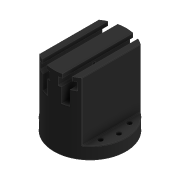
# Autodesk Inventor part: grippershape
Saved by Autodesk Inventor 2020.3 (Build 243373000, 373)
## iProperties
Created: 2020-05-25
Part Number: grippershape
Material: Generic
Document SubType Name: Modeling
Designer: Svend
Density: 1 g/cm^3
Appearance: Default
Author: Svend
Autodesk Inventor part; units mm, degrees
ref_plane "YZ Plane" through (0, 0, 0) normal (1, 0, 0) x (0, 1, 0)
ref_plane "XZ Plane" through (0, 0, 0) normal (0, 1, 0) x (-1, 0, 0)
ref_plane "XY Plane" through (0, 0, 0) normal (0, 0, 1) x (1, 0, 0)
ref_plane "Work Plane2" through (-6.6, -11, -70) normal (0, 0, -1) x (0, 1, 0)
ref_plane "Work Plane3" through (21.95, -1.9, -8.0264) normal (0, 0, 1) x (1, 0, 0)
ref_plane "Work Plane4" through (21.95, -1.9, -8.0264) normal (0, 0, 1) x (1, 0, 0)
sketch "Sketch3" plane through (21.95, -1.9, -8.0264) normal (0, 0, 1) x (1, 0, 0)
  line L0 (-6.75, 7.95) -> (-6.75, 1.35) projected
  line L1 (-6.75, 1.35) -> (-6.55, 1.15) projected
  line L2 (-6.55, 1.15) -> (-1.7, 1.15) projected
  line L3 (-1.7, 1.15) -> (-1.7, -12.85) projected
  line L4 (-4.0364, -12.85) -> (-4.0294, -12.85) projected
  line L5 (-2.65, -12.85) -> (-4.0294, -12.85) projected
  line L6 (-1.7, -12.85) -> (-2.65, -12.85) projected
  line L7 (-2.65, -12.85) -> (-2.65, -0.85) projected
  line L8 (-6.75, 7.95) -> (-6.55, 8.15) projected
  line L9 (-3.2, 8.15) -> (-6.55, 8.15) projected
  line L10 (-3.2, 12.75) -> (-3.2, 8.15) projected
  line L11 (-3.2, 12.75) -> (-3, 12.95) projected
  line L12 (3.1, 12.95) -> (-3, 12.95) projected
  line L13 (3.1, 12.95) -> (3.3, 12.75) projected
  line L14 (3.3, 8.15) -> (3.3, 12.75) projected
  line L15 (6.65, 8.15) -> (3.3, 8.15) projected
  line L16 (6.65, 8.15) -> (6.85, 7.95) projected
  line L17 (6.85, 1.35) -> (6.85, 7.95) projected
  line L18 (6.85, 1.35) -> (6.65, 1.15) projected
  line L19 (1.8, 1.15) -> (6.65, 1.15) projected
  line L20 (1.8, -12.65) -> (1.8, 1.15) projected
  line L21 (1.8, -12.85) -> (1.8, -12.65) projected
  line L22 (-1.7, -12.85) -> (1.8, -12.85) projected
  line L23 (-4.0294, -12.85) -> (-4.125, 1.15)
  line L24 (-7.05, 1.2257) -> (-7.05, 8.0743)
  line L25 (-7.05, 8.0743) -> (-6.6743, 8.45)
  line L26 (-6.6743, 8.45) -> (-3.5, 8.45)
  line L27 (-3.5, 8.45) -> (-3.5, 12.8743)
  line L28 (-3.5, 12.8743) -> (-3.1243, 13.25)
  line L29 (-3.1243, 13.25) -> (3.2243, 13.25)
  line L30 (3.2243, 13.25) -> (3.6, 12.8743)
  line L31 (3.6, 12.8743) -> (3.6, 8.45)
  line L32 (3.6, 8.45) -> (6.7743, 8.45)
  line L33 (6.7743, 8.45) -> (7.15, 8.0743)
  line L34 (7.15, 8.0743) -> (7.15, 1.2257)
  line L35 (7.15, 1.2257) -> (6.7743, 0.85)
  line L36 (6.7743, 0.85) -> (2.1, 0.85)
  line L37 (2.1, 0.85) -> (2.1, -12.65)
  line L38 (2.1, -12.65) -> (2.1, -13.15)
  line L39 (2.1, -13.15) -> (-2, -13.15)
  line L40 (-2, -13.15) -> (-2, 0.85)
  line L41 (-2, 0.85) -> (-6.6743, 0.85)
  line L42 (-6.6743, 0.85) -> (-7.05, 1.2257)
  line L43 (-4.1273, -13.15) -> (-4.2253, 1.1991)
  line L44 (-2, -13.15) -> (-4.1273, -13.15)
  line L45 (-13.925, -1.05) -> (-8.025, -1.05) projected
  line L46 (-10.975, -1.05) -> (-10.975, -12.3939)
  line L47 (-15.2, 7.95) -> (-15.2, 1.35)
  line L48 (-15.2, 1.35) -> (-15.4, 1.15)
  line L49 (-15.4, 1.15) -> (-20.25, 1.15)
  line L50 (-20.25, 1.15) -> (-20.25, -12.85)
  line L51 (-17.9136, -12.85) -> (-17.9206, -12.85)
  line L52 (-19.3, -12.85) -> (-17.9206, -12.85)
  line L53 (-20.25, -12.85) -> (-19.3, -12.85)
  line L54 (-19.3, -12.85) -> (-19.3, -0.85)
  line L55 (-15.2, 7.95) -> (-15.4, 8.15)
  line L56 (-18.75, 8.15) -> (-15.4, 8.15)
  line L57 (-18.75, 12.75) -> (-18.75, 8.15)
  line L58 (-18.75, 12.75) -> (-18.95, 12.95)
  line L59 (-25.05, 12.95) -> (-18.95, 12.95)
  line L60 (-25.05, 12.95) -> (-25.25, 12.75)
  line L61 (-25.25, 8.15) -> (-25.25, 12.75)
  line L62 (-28.6, 8.15) -> (-25.25, 8.15)
  line L63 (-28.6, 8.15) -> (-28.8, 7.95)
  line L64 (-28.8, 1.35) -> (-28.8, 7.95)
  line L65 (-28.8, 1.35) -> (-28.6, 1.15)
  line L66 (-23.75, 1.15) -> (-28.6, 1.15)
  line L67 (-23.75, -12.65) -> (-23.75, 1.15)
  line L68 (-23.75, -12.85) -> (-23.75, -12.65)
  line L69 (-20.25, -12.85) -> (-23.75, -12.85)
  line L70 (-17.9206, -12.85) -> (-17.825, 1.15)
  line L71 (-14.9, 1.2257) -> (-14.9, 8.0743)
  line L72 (-14.9, 8.0743) -> (-15.2757, 8.45)
  line L73 (-15.2757, 8.45) -> (-18.45, 8.45)
  line L74 (-18.45, 8.45) -> (-18.45, 12.8743)
  line L75 (-18.45, 12.8743) -> (-18.8257, 13.25)
  line L76 (-18.8257, 13.25) -> (-25.1743, 13.25)
  line L77 (-25.1743, 13.25) -> (-25.55, 12.8743)
  line L78 (-25.55, 12.8743) -> (-25.55, 8.45)
  line L79 (-25.55, 8.45) -> (-28.7243, 8.45)
  line L80 (-28.7243, 8.45) -> (-29.1, 8.0743)
  line L81 (-29.1, 8.0743) -> (-29.1, 1.2257)
  line L82 (-29.1, 1.2257) -> (-28.7243, 0.85)
  line L83 (-28.7243, 0.85) -> (-24.05, 0.85)
  line L84 (-24.05, 0.85) -> (-24.05, -12.65)
  line L85 (-24.05, -12.65) -> (-24.05, -13.15)
  line L86 (-24.05, -13.15) -> (-19.95, -13.15)
  line L87 (-19.95, -13.15) -> (-19.95, 0.85)
  line L88 (-19.95, 0.85) -> (-15.2757, 0.85)
  line L89 (-15.2757, 0.85) -> (-14.9, 1.2257)
  line L90 (-17.8227, -13.15) -> (-17.7247, 1.1991)
  line L91 (-19.95, -13.15) -> (-17.8227, -13.15)
  line L92 (-33.425, 12.25) -> (11.575, 12.25)
  line L93 (11.575, 12.25) -> (11.575, -57.75)
  line L94 (11.575, -57.75) -> (-33.425, -57.75)
  line L95 (-33.425, -57.75) -> (-33.425, 12.25)
  point P0 (-21.95, 1.9)
  point P1 (-10.925, -52.6184)
  point P2 (-10.925, -57.75)
  point P3 (-3.5, 12.25)
  point P4 (-18.45, 12.25)
  point P5 (-17.727, 0.85)
  point P6 (-25.55, 12.25)
  point P7 (3.6, 12.25)
  point P8 (-4.223, 0.85)
  dimension "d18" = 0.3
  dimension "d19" = 0.1
  dimension "d20" = 1
  dimension "d21" = 45
  dimension "d22" = 70
  constraints: 144 end point, 45 symmetric about line, 3 midpoint, 3 parallel, 2 horizontal, 1 perpendicular, 1 vertical, 1 vertical alignment, 18 other
  measures "d18" distance between parallel lines of L0 L24
  measures "d19" distance between parallel lines of L23 L43
  measures "d20" distance between parallel lines of L76 L92
  measures "d21" distance of L93.end L94.end
  measures "d22" distance between parallel lines of L92 L94
extrude "Extrusion2" add sketch "Sketch3" against normal blind 70 contours L43 L44 L39 L38 L37 L36 L35 L34 L33 L32 L31 L92 L93 L94 L95 L78 L79 L80 L81 L82 L83 L84 L85 L86 L91 L90 L88 L89 L71 L72 L73 L74 L27 L26 L25 L24 L42 L41
sketch "Sketch4" plane through (-11.475, -59.65, -8.0264) normal (0, -1, 0) x (1, 0, 0)
  line L0 (0, 0) -> (45, 0) projected
  line L1 (0, 0) -> (0, -70) projected
  line L2 (45, -70) -> (0, -70) projected
  line L3 (45, 0) -> (45, -70) projected
  circle A0 centre (22.5, -35) radius 9
  point P0 (11.475, 8.0264)
  point P1 (22.5, 0)
  point P2 (45, -35)
  dimension "d25" = 18
  constraints: 2 midpoint, 1 centre point, 1 horizontal alignment, 1 vertical alignment
  measures "d25" diameter of A0
ref_plane "Work Plane5" through (1.75, -2.8, -26.5932) normal (0, 1, 0) x (0, 0, 1)
extrude "Extrusion3" cut sketch "Sketch4" against normal blind 57.25 contours A0
sketch "Sketch5" plane through (-11.475, -59.65, -8.0264) normal (0, -1, 0) x (1, 0, 0)
  circle A0 centre (22.5, -35) radius 9 projected
  circle A1 centre (22.5, -35) radius 4
  point P0 (11.475, 8.0264)
  dimension "d28" = 8
  constraints: 1 centre point, 1 coincident
  measures "d28" diameter of A1
extrude "Extrusion4" cut sketch "Sketch5" against normal blind 61 contours A1
ref_plane "Work Plane6" through (1.2787, -51.0682, -52.9264) normal (0, 0, -1) x (0, 1, 0)
sketch "Sketch8" plane through (-11.475, -59.65, -8.0264) normal (0, -1, 0) x (1, 0, 0)
  circle A0 centre (22.5, -35) radius 9 projected
  circle A1 centre (22.5, -35) radius 9 projected
  line L0 (0, 0) -> (45, 0) projected
  line L1 (0, 0) -> (0, -70) projected
  line L2 (45, -70) -> (0, -70) projected
  line L3 (45, 0) -> (45, -70) projected
  arc A2 (26.375, -34.0078) -> (18.525, -34.5535) centre (22.5, -35) ccw projected
  circle A3 centre (22.5, -35) radius 35
  point P0 (11.475, 8.0264)
  point P1 (45, -8.1905)
  point P2 (45, -61.8095)
  point P3 (0, -61.8095)
  point P4 (0, -8.1905)
  point P5 (22.5, -70)
  point P6 (22.5, 0)
  constraints: 1 centre point, 1 coincident, 1 tangent
extrude "Extrusion10" cut sketch "Sketch8" against normal through all contours L0 A3 L1 | L0 L3 A3 | A3 L2 L1 | L3 L2 A3
ref_plane "Work Plane7" through (10.975, -59.9, -43.0264) normal (0, -1, 0) x (1, 0, 0)
sketch "Sketch10" plane through (10.975, -59.9, -43.0264) normal (0, -1, 0) x (1, 0, 0)
  line L0 (29.6, 9.9) -> (-9, 9.9) projected
  arc A0 (-9, 9.9) -> (-10, 8.9) centre (-9, 8.9) ccw projected
  line L1 (-10, 8.9) -> (-10, -8.9) projected
  arc A1 (30.6, 8.9) -> (29.6, 9.9) centre (29.6, 8.9) ccw projected
  line L2 (30.6, -8.9) -> (30.6, 8.9) projected
  arc A2 (29.6, -9.9) -> (30.6, -8.9) centre (29.6, -8.9) ccw projected
  line L3 (-9, -9.9) -> (29.6, -9.9) projected
  arc A3 (-10, -8.9) -> (-9, -9.9) centre (-9, -8.9) ccw projected
  line L4 (-10, 8.9) -> (-10, -8.9) projected
  line L5 (-10.2, -12) -> (-10.2, 30.5)
  line L6 (-10.2, 30.5) -> (10.2, 30.5)
  line L7 (10.2, 30.5) -> (10.2, -12)
  line L8 (10.2, -12) -> (-10.2, -12)
  circle A4 centre (0, 0) radius 9 projected
  circle A5 centre (0.05, 0) radius 9 projected
  arc A6 (22.55, 26.8095) -> (-22.45, 26.8095) centre (0.05, 0) ccw projected
  line L9 (-22.45, 26.8095) -> (-22.45, -26.8095) projected
  arc A7 (-22.45, -26.8095) -> (22.55, -26.8095) centre (0.05, 0) ccw projected
  line L10 (22.55, 26.8095) -> (22.55, -26.8095) projected
  point P0 (-10.975, 43.0264)
  point P1 (0, -12)
  dimension "d45" = 20.4
  dimension "d46" = 12
  dimension "d47" = 30.5
  constraints: 8 end point, 2 parallel, 1 midpoint, 1 perpendicular
  measures "d45" distance between parallel lines of L7 L5
  measures "d46" distance from line of L8 A4.centre
  measures "d47" distance from line of L6 A4.centre
extrude "Extrusion12" cut sketch "Sketch10" against normal blind 43 contours L7 L3 A3 L1 A0 L0 | L0 A0 L1 A3 L3 L7 L8 L5 L6 | A4 A5 | A4 A5 | A5 A4
sketch "Sketch11" plane through (0.775, -59.65, -55.0264) normal (0, 0, 1) x (1, 0, 0)
  line L0 (20.4, 0) -> (0, 0) projected
  line L1 (20.4, 0) -> (20.4, 42.75) projected
  line L2 (20.4, 42.75) -> (0, 42.75) projected
  line L3 (0, 0) -> (0, 42.75) projected
  line L4 (5.7, 15) -> (14.7, 15)
  line L5 (14.7, 15) -> (14.7, 8)
  line L6 (14.7, 8) -> (5.7, 8)
  line L7 (5.7, 8) -> (5.7, 15)
  point P0 (-32.8264, 59.9)
  point P1 (10.2, 8)
  point P2 (10.2, 0)
  dimension "d50" = 8
  dimension "d51" = 7
  dimension "d52" = 9
  constraints: 8 end point, 2 midpoint, 2 parallel, 1 horizontal, 1 perpendicular, 1 vertical alignment
  measures "d50" distance between parallel lines of L0 L6
  measures "d51" distance between parallel lines of L6 L4
  measures "d52" distance between parallel lines of L7 L5
extrude "Extrusion13" cut sketch "Sketch11" against normal through all contours L4 L5 L6 L7
fillet "Fillet10" radius 0.2 4 edges at (25.55, 10.35, -43.0264) (18.45, 10.35, -43.0264) (3.5, 10.35, -43.0264) (-3.6, 10.35, -43.0264)
chamfer "Chamfer5" distance 0.5 angle 45 6 edges at (20.0062, -15.05, -42.4455) (20.0062, -15.05, -43.6074) (19.2357, -15.05, -39.3407) (19.2357, -15.05, -46.7122) (2.025, -15.05, -43.0264) (7.025, -2.4, -43.0264)
fillet "Fillet11" radius 0.2 10 edges at (4.1256, -15.3001, -37.2473) (4.1703, -8.7525, -37.1943) (4.2137, -2.4, -43.0264) (4.1256, -15.3001, -48.8056) (4.1703, -8.7525, -48.8586) (17.7796, -8.7511, -48.9741) (17.8244, -15.3001, -48.9229) (17.7363, -2.4, -43.0264) (17.8244, -15.3001, -37.13) (17.7796, -8.7511, -37.0788)
extrude "Extrusion14" add sketch "Sketch8" against normal blind 13.15 contours L1 A3 | A3 L3
sketch "Sketch13" plane through (11.025, 10.35, -43.0264) normal (0, 1, 0) x (0.9999989, 0, 0.0014605)
  circle A0 centre (0, 0) radius 35 projected
  line L0 (22.5391, -26.7766) -> (22.4608, 26.8423) projected
  line L1 (-22.5391, 26.7766) -> (-22.4608, -26.8423) projected
  line L2 (20.5414, -28.3381) -> (20.4585, 28.398)
  arc A1 (22.4608, 26.8423) -> (14.6786, 31.7732) centre (0, 0) ccw projected
  arc A2 (-14.8713, 31.6835) -> (-22.5391, 26.7766) centre (0, 0) ccw projected
  line L3 (-20.5, 28.3681) -> (-20.5, -28.3681)
  point P0 (-10.9621, -43.0425)
  point P1 (20.4585, 28.398)
  dimension "d85" = 2
  dimension "d86" = 2
  constraints: 4 end point, 2 point on circle, 1 parallel, 1 vertical, 4 other
  measures "d85" distance between parallel lines of L0 L2
extrude "Extrusion15" cut sketch "Sketch13" against normal up to surface (56.85 mm away) contours L0 A0 L2 | A0 L1 L3
sketch "Sketch14" plane through (11.025, -59.65, -43.0264) normal (0, -1, 0) x (1, 0, 0)
  line L0 (10.15, -12) -> (-10.25, -12) projected
  line L1 (-10.25, -12) -> (-10.25, 30.5) projected
  line L2 (-10.25, 30.5) -> (10.15, 30.5) projected
  line L3 (10.15, 30.5) -> (10.15, -12) projected
  circle A0 centre (0, 0) radius 35 projected
  circle A1 centre (28, 0) radius 2.1
  arc A2 (-9, 0) -> (-9, 0) centre (0, 0) ccw projected
  circle A3 centre (24.2487, 14) radius 2.1
  circle A4 centre (14, 24.2487) radius 2.1
  circle A5 centre (0, 28) radius 2.1
  circle A6 centre (-14, 24.2487) radius 2.1
  circle A7 centre (-24.2487, 14) radius 2.1
  circle A8 centre (-28, 0) radius 2.1
  circle A9 centre (-24.2487, -14) radius 2.1
  circle A10 centre (-14, -24.2487) radius 2.1
  circle A11 centre (0, -28) radius 2.1
  circle A12 centre (14, -24.2487) radius 2.1
  circle A13 centre (24.2487, -14) radius 2.1
  point P0 (-11.025, 43.0264)
  dimension "d89" = 28
  dimension "d90" = 4.2
  dimension "d93" = 360
  constraints: 12 centre point, 1 horizontal alignment, 25 other
  measures "d89" distance of A2.centre A1.centre
  measures "d90" diameter of A1
extrude "Extrusion16" cut sketch "Sketch14" against normal through all contours A1 | A3 | A7 | A8 | A9 | A13
sketch "Sketch15" plane through (11.025, -59.65, -43.0264) normal (0, -1, 0) x (1, 0, 0)
  circle A0 centre (24.2487, -14) radius 2.1 projected
  circle A1 centre (-24.2487, 14) radius 2.1 projected
  circle A2 centre (28, 0) radius 2.1 projected
  circle A3 centre (-24.2487, -14) radius 2.1 projected
  circle A4 centre (-28, 0) radius 2.1 projected
  circle A5 centre (24.2487, 14) radius 2.1 projected
  line L0 (10.15, -12) -> (-10.25, -12) projected
  line L1 (-10.25, -12) -> (-10.25, 30.5) projected
  line L2 (-10.25, 30.5) -> (10.15, 30.5) projected
  line L3 (10.15, 30.5) -> (10.15, -12) projected
  circle A6 centre (0, 0) radius 35 projected
  point P0 (-11.025, 43.0264)
extrude "Extrusion17" cut sketch "Sketch15" against normal blind 1.15
fillet "Fillet12" radius 0.5 48 edges at (11.025, -58.5, -8.0264) (11.025, -58.5, -78.0264) (-23.975, -58.5, -43.0264) (46.025, -58.5, -43.0264) (33.1737, -58.5, -29.0264) (36.925, -58.5, -43.0264) (33.1737, -58.5, -57.0264) (-15.3237, -58.5, -57.0264) (-19.075, -58.5, -43.0264) (-15.3237, -58.5, -29.0264) (-10.5093, -46.5, -15.4352) (-10.469, -46.5, -70.6491) (-23.975, -46.5, -43.0264) (-11.2135, -46.5, -28.4191) (-11.2135, -46.5, -29.6338) (-15.3237, -46.5, -29.0264) (-19.075, -46.5, -43.0264) (-11.2135, -46.5, -56.4191) (-11.2135, -46.5, -57.6338) (-15.3237, -46.5, -57.0264) (-9.475, -46.5, -43.0564) (21.175, -58.5, -33.7764) (10.975, -58.5, -55.0264) (0.775, -58.5, -33.7764) (10.975, -58.5, -12.5264) (31.525, -46.5, -43.0264) (33.1737, -46.5, -29.0264) (35.881, -46.5, -31.0367) (35.881, -46.5, -27.0162) (36.925, -46.5, -43.0264) (33.1737, -46.5, -57.0264) (35.881, -46.5, -59.0367) (35.881, -46.5, -55.0162) (32.5391, -46.5, -15.4195) (32.5391, -46.5, -70.6334) (46.025, -46.5, -43.0264) (31.525, -18.075, -14.6583) (31.525, -18.075, -71.3946) (31.525, 10.35, -43.0264) (-9.475, 10.35, -43.0564) (-9.5164, -18.075, -14.6883) (-9.4335, -18.075, -71.4245) (10.975, -44.65, -55.0264) (10.975, -51.65, -55.0264) (10.9746, -44.65, -78.0264) (6.475, -48.15, -77.7294) (15.475, -48.15, -77.7424) (10.9746, -51.65, -78.0264)
sketch "Sketch16" plane through (11.025, -58.5, -43.0264) normal (0, -1, 0) x (1, 0, 0)
  arc A0 (-4.5549, -34.198) -> (4.4547, -34.2112) centre (0, 0) ccw projected
  arc A1 (4.45, -34.143) -> (4.4547, -34.2112) centre (4.95, -34.143) ccw projected
  line L0 (4.45, -12.5) -> (4.45, -34.143) projected
  line L1 (-4.55, -12.5) -> (4.45, -12.5) projected
  line L2 (-4.55, -12.5) -> (-4.55, -34.1284) projected
  arc A2 (-4.5549, -34.198) -> (-4.55, -34.1284) centre (-5.05, -34.1284) ccw projected
  line L3 (10.15, -12) -> (-10.25, -12) projected
  line L4 (-4.55, -12.5) -> (-4.55, -34.1284) projected
  line L5 (4.45, -12) -> (-4.55, -12)
  line L6 (-4.55, -12) -> (-4.55, -27)
  line L7 (-4.55, -27) -> (4.45, -27)
  line L8 (4.45, -27) -> (4.45, -12)
  point P0 (-11.025, 43.0264)
  point P1 (-4.55, -27)
  point P2 (4.45, -27)
  point P3 (4.45, -12.5)
  point P4 (-4.55, -12)
  dimension "d100" = 15
  constraints: 8 end point, 2 collinear, 2 parallel, 2 point on line, 1 horizontal, 1 perpendicular
  measures "d100" distance of L6.end L5.end
extrude "Extrusion18" cut sketch "Sketch16" against normal up to surface (13.85 mm away) contours L2 L1 L0 L7 | L6 L3 L8 L1
sketch "Sketch17" plane through (11.025, -58.5, -43.0264) normal (0, -1, 0) x (1, 0, 0)
  line L0 (4.45, -12.5) -> (4.45, -27) projected
  line L1 (4.45, -27) -> (-4.55, -27) projected
  line L2 (-4.55, -27) -> (-4.55, -12.5) projected
  line L3 (-10.75, -12.5) -> (-4.55, -12.5) projected
  line L4 (-10.75, 31) -> (-10.75, -12.5) projected
  line L5 (10.65, 31) -> (-10.75, 31) projected
  line L6 (10.65, -12.5) -> (10.65, 31) projected
  line L7 (4.45, -12.5) -> (10.65, -12.5) projected
  circle A0 centre (-28, 0) radius 2.6 projected
  circle A1 centre (24.2487, -14) radius 2.6 projected
  circle A2 centre (24.2487, 14) radius 2.6 projected
  circle A3 centre (0, 0) radius 34.5 projected
  circle A4 centre (28, 0) radius 2.6 projected
  circle A5 centre (-24.2487, -14) radius 2.6 projected
  circle A6 centre (-24.2487, 14) radius 2.6 projected
  line L8 (-10.75, -12.5) -> (-4.55, -12.5) projected
  line L9 (5.95, -35) -> (-6.05, -35)
  line L10 (-6.05, -35) -> (-6.05, -12.5)
  line L11 (-6.05, -12.5) -> (5.95, -12.5)
  line L12 (5.95, -12.5) -> (5.95, -35)
  circle A7 centre (0, 0) radius 35 projected
  line L13 (7.7, -29.2) -> (-7.7, -29.2)
  line L14 (-7.7, -29.2) -> (-7.7, -27)
  line L15 (-7.7, -27) -> (7.7, -27)
  line L16 (7.7, -27) -> (7.7, -29.2)
  line L17 (10.15, -12) -> (4.45, -12) projected
  line L18 (4.45, -12) -> (-4.55, -12) projected
  line L19 (-4.55, -12) -> (-10.25, -12) projected
  line L20 (5.95, -12.5) -> (5.95, -12)
  line L21 (-6.05, -12.5) -> (-6.05, -12)
  point P0 (-11.025, 43.0264)
  point P1 (-0.05, -35)
  point P2 (-0.05, -27)
  point P3 (0, -29.2)
  point P4 (-6.05, -29.2)
  point P5 (-6.05, -33.9654)
  point P6 (5.95, -33.983)
  point P7 (5.95, -29.2)
  point P8 (5.95, -27)
  point P9 (-6.05, -27)
  point P10 (5.95, -34.4905)
  point P11 (-6.05, -34.4731)
  dimension "d104" = 12
  dimension "d105" = 15.4
  dimension "d106" = 2.2
  constraints: 20 end point, 4 parallel, 4 perpendicular, 3 midpoint, 3 point on line, 2 horizontal, 2 vertical alignment, 1 collinear, 1 tangent
  measures "d104" distance between parallel lines of L12 L10
  measures "d105" distance between parallel lines of L16 L14
  measures "d106" distance between parallel lines of L1 L13
extrude "Extrusion19" cut sketch "Sketch17" against normal blind 15.5 contours L7 L12 L15 L0 | L11 L3 L21 L19 L18 L17 L20 L7 | L0 L1 L2 L11 | L15 L12 L13 L10 L1 | L2 L15 L10 L3 | L15 L16 L13 L12 | L10 L13 L14 L15 | L12 A3 L10 L13 | L12 A7 L10 A3 picked at (3.9619, -34.4002)
sketch "Sketch18" plane through (0.775, -16.9, -55.0264) normal (0, 0, 1) x (1, 0, 0)
  line L0 (4.2, -41.1) -> (4.2, -26.1) projected
  line L1 (4.2, -26.1) -> (16.2, -26.1) projected
  line L2 (16.2, -26.1) -> (16.2, -41.1) projected
  arc A0 (16.2, -33.6) -> (4.2, -33.6) centre (10.2, -33.6) ccw
  point P0 (-0.775, 16.9)
  constraints: 2 midpoint, 2 point on circle, 2 tangent, 1 centre point
extrude "Extrusion20" add sketch "Sketch18" against normal up to surface (15 mm away)
sketch "Sketch19" plane through (3.325, -58.5, -72.2264) normal (0, 0, 1) x (1, 0, 0)
  line L0 (0, 0) -> (1.65, 0) projected
  line L1 (0, 0) -> (0, 15.5) projected
  line L2 (0, 15.5) -> (15.4, 15.5) projected
  line L3 (15.4, 0) -> (15.4, 15.5) projected
  line L4 (13.65, 0) -> (15.4, 0) projected
  line L5 (13.65, 0) -> (13.65, 8) projected
  arc A0 (13.65, 8) -> (1.65, 8) centre (7.65, 8) ccw projected
  line L6 (1.65, 0) -> (1.65, 8) projected
  line L7 (-1.1, 8) -> (-1.1, 0)
  line L8 (42.2, 0) -> (-26.8, 0) projected
  line L9 (16.4, 8) -> (16.4, 0)
  arc A1 (16.4, 8) -> (-1.1, 8) centre (7.65, 8) ccw
  point P0 (-3.325, 58.5)
  point P1 (15.4, 12.062)
  point P2 (0, 12.2474)
  point P3 (16.4, 0)
  constraints: 4 end point, 2 point on circle, 2 tangent, 2 vertical, 1 centre point, 1 coincident, 1 point on line
extrude "Extrusion21" cut sketch "Sketch19" against normal up to surface contours L1 A1 L2 L3 L4 L5 A0 L6 L0 | L8 L7 A1 L1 | A1 L2 | L3 A1 L9 L8 round surface about axis through (11.025, -59.65, -43.0264) along (0, 1, 0) radius 35 far side no
sketch "Sketch20" plane through (16.975, -43, -72.2264) normal (0, 0, 1) x (1, 0, 0)
  line L0 (0, -1.1311) -> (0, 0) projected
  line L1 (0, 0) -> (-1.4931, 0) projected
  line L2 (-10.5069, 0) -> (-12, 0) projected
  line L3 (-12, 0) -> (-12, -1.1311) projected
  line L4 (2.75, -15) -> (-14.75, -15) projected
  line L5 (8.775, 53.35) -> (14.05, 53.35) projected
  line L6 (8.575, 49.55) -> (8.575, 53.15) projected
  line L7 (11.7493, 49.55) -> (8.575, 49.55) projected
  line L8 (12.125, 49.1743) -> (11.7493, 49.55) projected
  line L9 (12.125, 42.3257) -> (12.125, 49.1743) projected
  line L10 (11.7493, 41.95) -> (12.125, 42.3257) projected
  line L11 (7.075, 41.95) -> (11.7493, 41.95) projected
  line L12 (7.075, 27.95) -> (7.075, 41.95) projected
  line L13 (0.8477, 27.95) -> (7.075, 27.95) projected
  line L14 (0.752, 41.95) -> (0.8477, 27.95) projected
  line L15 (-1.6993, 41.95) -> (0.752, 41.95) projected
  line L16 (-2.075, 42.3257) -> (-1.6993, 41.95) projected
  line L17 (-2.075, 49.1743) -> (-2.075, 42.3257) projected
  line L18 (-1.6993, 49.55) -> (-2.075, 49.1743) projected
  line L19 (1.475, 49.55) -> (-1.6993, 49.55) projected
  line L20 (1.475, 53.15) -> (1.475, 49.55) projected
  line L21 (-13.275, 53.35) -> (1.275, 53.35) projected
  line L22 (-13.475, 49.55) -> (-13.475, 53.15) projected
  line L23 (-10.3007, 49.55) -> (-13.475, 49.55) projected
  line L24 (-9.925, 49.1743) -> (-10.3007, 49.55) projected
  line L25 (-9.925, 42.3257) -> (-9.925, 49.1743) projected
  line L26 (-10.3007, 41.95) -> (-9.925, 42.3257) projected
  line L27 (-12.752, 41.95) -> (-10.3007, 41.95) projected
  line L28 (-12.8477, 27.95) -> (-12.752, 41.95) projected
  line L29 (-19.075, 27.95) -> (-12.8477, 27.95) projected
  line L30 (-19.075, 41.95) -> (-19.075, 27.95) projected
  line L31 (-23.7493, 41.95) -> (-19.075, 41.95) projected
  line L32 (-24.125, 42.3257) -> (-23.7493, 41.95) projected
  line L33 (-24.125, 49.1743) -> (-24.125, 42.3257) projected
  line L34 (-23.7493, 49.55) -> (-24.125, 49.1743) projected
  line L35 (-20.575, 49.55) -> (-23.7493, 49.55) projected
  line L36 (-20.575, 53.15) -> (-20.575, 49.55) projected
  line L37 (-25.9919, 53.35) -> (-20.775, 53.35) projected
  line L38 (-26.2815, -3) -> (-26.2815, 53.2574) projected
  line L39 (-27.2138, -4) -> (-27.2949, -4) projected
  line L40 (-26.1982, 53.2574) -> (-26.1982, -3) projected
  line L41 (-20.775, 53.35) -> (-25.908, 53.35) projected
  line L42 (-20.575, 49.55) -> (-20.575, 53.15) projected
  line L43 (-23.7493, 49.55) -> (-20.575, 49.55) projected
  line L44 (-24.125, 49.1743) -> (-23.7493, 49.55) projected
  line L45 (-24.125, 42.3257) -> (-24.125, 49.1743) projected
  line L46 (-23.7493, 41.95) -> (-24.125, 42.3257) projected
  line L47 (-19.075, 41.95) -> (-23.7493, 41.95) projected
  line L48 (-19.075, 27.95) -> (-19.075, 41.95) projected
  line L49 (-12.8477, 27.95) -> (-19.075, 27.95) projected
  line L50 (-12.752, 41.95) -> (-12.8477, 27.95) projected
  line L51 (-10.3007, 41.95) -> (-12.752, 41.95) projected
  line L52 (-9.925, 42.3257) -> (-10.3007, 41.95) projected
  line L53 (-9.925, 49.1743) -> (-9.925, 42.3257) projected
  line L54 (-10.3007, 49.55) -> (-9.925, 49.1743) projected
  line L55 (-13.475, 49.55) -> (-10.3007, 49.55) projected
  line L56 (-13.475, 53.15) -> (-13.475, 49.55) projected
  line L57 (1.275, 53.35) -> (-13.275, 53.35) projected
  line L58 (1.475, 49.55) -> (1.475, 53.15) projected
  line L59 (-1.6993, 49.55) -> (1.475, 49.55) projected
  line L60 (-2.075, 49.1743) -> (-1.6993, 49.55) projected
  line L61 (-2.075, 42.3257) -> (-2.075, 49.1743) projected
  line L62 (-1.6993, 41.95) -> (-2.075, 42.3257) projected
  line L63 (0.752, 41.95) -> (-1.6993, 41.95) projected
  line L64 (0.8477, 27.95) -> (0.752, 41.95) projected
  line L65 (7.075, 27.95) -> (0.8477, 27.95) projected
  line L66 (7.075, 41.95) -> (7.075, 27.95) projected
  line L67 (11.7493, 41.95) -> (7.075, 41.95) projected
  line L68 (12.125, 42.3257) -> (11.7493, 41.95) projected
  line L69 (12.125, 49.1743) -> (12.125, 42.3257) projected
  line L70 (11.7493, 49.55) -> (12.125, 49.1743) projected
  line L71 (8.575, 49.55) -> (11.7493, 49.55) projected
  line L72 (8.575, 53.15) -> (8.575, 49.55) projected
  line L73 (14.05, 53.35) -> (8.775, 53.35) projected
  line L74 (14.3399, -3) -> (14.3399, 53.2574) projected
  line L75 (15.3543, -4) -> (15.3543, -4) projected
  line L76 (14.3399, 53.2574) -> (14.3399, -3) projected
  circle A0 centre (-6, -7.5) radius 8.75
  line L77 (2.75, -15) -> (2.75, -7.5) projected
  line L78 (-14.75, -7.5) -> (-14.75, -15) projected
  point P0 (-16.975, 43)
  point P1 (-10.5069, 0)
  point P2 (-1.4931, 0)
  point P3 (0, -1.1311)
  constraints: 1 centre point, 1 horizontal alignment, 20 other
extrude "Extrusion22" add sketch "Sketch20" against normal up to surface contours A0 L1 L0 | A0 L3 L2 round surface about axis through (11.025, -59.65, -43.0264) along (0, 1, 0) radius 35 far side no
sketch "Sketch21" plane through (11.025, -43, -43.0264) normal (0, -1, 0) x (1, 0, 0)
  line L0 (-4.5569, -29.2) -> (-7.7, -29.2) projected
  line L1 (-4.5569, -29.2) -> (4.4569, -29.2) projected
  line L2 (4.4569, -29.2) -> (7.7, -29.2) projected
  line L3 (7.7, -27) -> (7.7, -29.2) projected
  line L4 (-7.7, -27) -> (7.7, -27) projected
  line L5 (-7.7, -29.2) -> (-7.7, -27) projected
  point P0 (-11.025, 43.0264)
extrude "Extrusion23" cut sketch "Sketch21" against normal blind 3
fillet "Fillet14" radius 7.7 2 edges at (3.325, -40, -71.1264) (18.725, -40, -71.1264)
sketch "Sketch22" plane through (3.325, -58.5, -72.2264) normal (0, 0, -1) x (-1, 0, 0)
  arc A0 (0, 10.8) -> (-15.4, 10.8) centre (-7.7, 10.8) ccw projected
  line L0 (-15.4, 0) -> (-15.4, 10.8) projected
  line L1 (-13.65, 0) -> (-15.4, 0) projected
  line L2 (-13.65, 0) -> (-13.65, 8) projected
  arc A1 (-1.65, 8) -> (-13.65, 8) centre (-7.65, 8) ccw projected
  line L3 (-1.65, 0) -> (-1.65, 8) projected
  line L4 (0, 0) -> (-1.65, 0) projected
  line L5 (0, 0) -> (0, 10.8) projected
  arc A2 (-0.2176, 12.6175) -> (-15.2425, 12.3492) centre (-7.65, 8) ccw projected
  line L6 (-15.4, 0) -> (-15.4, 10.8) projected
  arc A3 (-15.2425, 12.3492) -> (-15.4, 10.8) centre (-7.7, 10.8) ccw projected
  arc A4 (-15.2425, 12.3492) -> (-16.4, 8) centre (-7.65, 8) ccw projected
  line L7 (-16.4, 0) -> (-16.4, 8) projected
  line L8 (-15.4, 0) -> (-16.4, 0) projected
  line L9 (0, 0) -> (0, 10.8) projected
  line L10 (1.1, 0) -> (0, 0) projected
  line L11 (1.1, 8) -> (1.1, 0) projected
  arc A5 (1.1, 8) -> (-0.2176, 12.6175) centre (-7.65, 8) ccw projected
  arc A6 (0, 10.8) -> (-0.2176, 12.6175) centre (-7.7, 10.8) ccw projected
  point P0 (3.325, 58.5)
  point P1 (-0.2176, 12.6175)
  point P2 (-15.2425, 12.3492)
extrude "Extrusion24" add sketch "Sketch22" along normal blind 2.75
fillet "Fillet16" radius 0.2 37 edges at (4.975, -54.5, -72.2264) (16.975, -54.5, -72.2264) (10.975, -44.5, -72.2264) (4.975, -54.5, -74.9764) (16.975, -54.5, -74.9764) (10.975, -44.5, -74.9764) (10.975, -44.5, -70.0264) (4.975, -54.5, -70.0264) (16.975, -54.5, -70.0264) (16.2729, -43.5362, -77.6308) (10.9779, -41.75, -78.0264) (5.6771, -43.5362, -77.6155) (2.4969, -48.3359, -76.9716) (4.0499, -45.1515, -77.3244) (2.225, -54.25, -76.9021) (2.225, -58.3542, -76.7501) (2.225, -58.5, -75.6808) (19.725, -54.25, -76.9279) (19.725, -58.3541, -76.7761) (19.725, -58.5, -75.694) (17.9663, -45.2384, -77.3312) (19.4776, -48.4341, -76.9904) (3.6, -58.5, -74.9764) (18.35, -58.5, -74.9764) (17.85, -58.5, -72.2264) (18.725, -58.5, -71.1264) (17.85, -58.5, -70.0264) (4.15, -58.5, -70.0264) (3.325, -58.5, -71.1264) (4.15, -58.5, -72.2264) (4.975, -58.3536, -55.1729) (4.975, -54.25, -55.0264) (10.975, -44.5, -55.0264) (16.975, -54.25, -55.0264) (16.975, -58.3536, -55.1729) (16.975, -58.5, -62.7764) (4.975, -58.5, -62.7764)
body "Solid2"
